Autodesk Fusion 360 part; units mm, degrees
note: some values were not read from the file. Set by a fixed rule: which sketch regions a step uses.
(part 7 of 7)
  spline S19 degree 5 poles (3.4043, 3.4422) (3.4043, 3.4423) (3.4044, 3.4423) (3.4045, 3.4425) (3.4047, 3.4427) (3.405, 3.443) (3.4054, 3.4433) (3.4058, 3.4437) (3.4063, 3.4441) (3.4068, 3.4446) (3.4073, 3.4451) (3.4079, 3.4457) (3.4085, 3.4462) (3.4092, 3.4469) (3.41, 3.4475) (3.4107, 3.4482) (3.4116, 3.449) (3.4124, 3.4497) (3.4134, 3.4505) (3.4143, 3.4514) (3.4153, 3.4523) (3.4164, 3.4532) (3.4175, 3.4541) (3.4187, 3.4551) (3.4199, 3.4561) (3.4211, 3.4571) (3.4224, 3.4582) (3.4237, 3.4593) (3.4251, 3.4604) (3.4265, 3.4616) (3.428, 3.4628) (3.4295, 3.464) (3.4311, 3.4652) (3.4327, 3.4665) (3.4344, 3.4678) (3.4361, 3.4691) (3.4378, 3.4705) (3.4396, 3.4718) (3.4414, 3.4732) (3.4433, 3.4747) (3.4453, 3.4761) (3.4472, 3.4776) (3.4492, 3.4791) (3.4513, 3.4806) (3.4534, 3.4821) (3.4556, 3.4837) (3.4577, 3.4852) (3.46, 3.4868) (3.4623, 3.4885) (3.4646, 3.4901) (3.467, 3.4918) (3.4694, 3.4934) (3.4718, 3.4951) (3.4743, 3.4968) (3.4769, 3.4986) (3.4795, 3.5003) (3.4821, 3.5021) (3.4848, 3.5039) (3.4875, 3.5057) (3.4903, 3.5075) (3.4931, 3.5093) (3.4959, 3.5112) (3.4988, 3.513) (3.5018, 3.5149) (3.5047, 3.5168) (3.5078, 3.5187) (3.5108, 3.5206) (3.5139, 3.5225) (3.5171, 3.5244) (3.5203, 3.5264) (3.5235, 3.5284) (3.5268, 3.5303) (3.5301, 3.5323) (3.5335, 3.5343) (3.5369, 3.5363) (3.5403, 3.5383) (3.5438, 3.5404) (3.5473, 3.5424) (3.5509, 3.5444) (3.5545, 3.5465) (3.5582, 3.5486) (3.5619, 3.5506) (3.5656, 3.5527) (3.5694, 3.5548) (3.5732, 3.5569) (3.577, 3.559) (3.5809, 3.5611) (3.5849, 3.5632) (3.5889, 3.5653) (3.5929, 3.5674) (3.5969, 3.5696) (3.6011, 3.5717) (3.6052, 3.5738) (3.6094, 3.576) (3.6136, 3.5781) (3.6179, 3.5803) (3.6222, 3.5824) (3.6265, 3.5846) (3.6309, 3.5868) (3.6353, 3.5889) (3.6398, 3.5911) (3.6443, 3.5933) (3.6488, 3.5954) (3.6534, 3.5976) (3.658, 3.5998) (3.6627, 3.602) (3.6674, 3.6041) (3.6721, 3.6063) (3.6769, 3.6085) (3.6817, 3.6107) (3.6865, 3.6129) (3.6914, 3.615) (3.6964, 3.6172) (3.7013, 3.6194) (3.7063, 3.6216) (3.7114, 3.6238) (3.7165, 3.6259) (3.7216, 3.6281) (3.7267, 3.6303) (3.7319, 3.6324) (3.7372, 3.6346) (3.7424, 3.6368) (3.7477, 3.6389) (3.7531, 3.6411) (3.7585, 3.6433) (3.7639, 3.6454) (3.7693, 3.6476) (3.7748, 3.6497) (3.7803, 3.6518) (3.7859, 3.654) (3.7915, 3.6561) (3.7972, 3.6582) (3.8028, 3.6604) (3.8085, 3.6625) (3.8143, 3.6646) (3.8201, 3.6667) (3.8259, 3.6688) (3.8317, 3.6709) (3.8376, 3.673) (3.8436, 3.675) (3.8495, 3.6771) (3.8555, 3.6792) (3.8615, 3.6812) (3.8676, 3.6833) (3.8737, 3.6853) (3.8799, 3.6874) (3.886, 3.6894) (3.8922, 3.6914) (3.8985, 3.6934) (3.9048, 3.6954) (3.9111, 3.6974) (3.9174, 3.6994) (3.9238, 3.7014) (3.9302, 3.7034) (3.9366, 3.7053) (3.9431, 3.7073) (3.9496, 3.7092) (3.9562, 3.7112) (3.9628, 3.7131) (3.9694, 3.715) (3.976, 3.7169) (3.9827, 3.7188) (3.9894, 3.7207) (3.9962, 3.7225) (4.003, 3.7244) (4.0098, 3.7262) (4.0166, 3.7281) (4.0235, 3.7299) (4.0304, 3.7317) (4.0374, 3.7335) (4.0444, 3.7353) (4.0514, 3.7371) (4.0584, 3.7388) (4.0655, 3.7406) (4.0726, 3.7423) (4.0797, 3.744) (4.0869, 3.7457) (4.0941, 3.7474) (4.1013, 3.7491) (4.1086, 3.7508) (4.1159, 3.7524) (4.1232, 3.7541) (4.1306, 3.7557) (4.138, 3.7573) (4.1454, 3.7589) (4.1528, 3.7605) (4.1603, 3.7621) (4.1678, 3.7636) (4.1754, 3.7652) (4.1829, 3.7667) (4.1905, 3.7682) (4.1982, 3.7697) (4.2058, 3.7712) (4.2135, 3.7727) (4.2212, 3.7741) (4.229, 3.7755) (4.2368, 3.7769) (4.2446, 3.7783) (4.2524, 3.7797) (4.2603, 3.7811) (4.2682, 3.7825) (4.2761, 3.7838) (4.2841, 3.7851) (4.2921, 3.7864) (4.3001, 3.7877) (4.3081, 3.789) (4.3162, 3.7902) (4.3243, 3.7914) (4.3324, 3.7926) (4.3406, 3.7938) (4.3488, 3.795) (4.357, 3.7962) (4.3652, 3.7973) (4.3735, 3.7984) (4.3818, 3.7995) (4.3901, 3.8006) (4.3984, 3.8017) (4.4068, 3.8027) (4.4152, 3.8038) (4.4236, 3.8048) (4.4321, 3.8058) (4.4406, 3.8067) (4.4491, 3.8077) (4.4576, 3.8086) (4.4662, 3.8095) (4.4748, 3.8104) (4.4834, 3.8113) (4.4921, 3.8122) (4.5007, 3.813) (4.5094, 3.8138) (4.5181, 3.8146) (4.5269, 3.8154) (4.5357, 3.8161) (4.5445, 3.8169) (4.5533, 3.8176) (4.5621, 3.8183) (4.571, 3.8189) (4.5799, 3.8196) (4.5888, 3.8202) (4.5978, 3.8208) (4.6067, 3.8214) (4.6139, 3.8218) (4.6194, 3.8222) (4.623, 3.8224) (4.6248, 3.8225) knots 0 0 0 0 0 0 0.00416667 0.00833333 0.0125 0.01666667 0.02083333 0.025 0.02916667 0.03333333 0.0375 0.04166667 0.04583333 0.05 0.05416667 0.05833333 0.0625 0.06666667 0.07083333 0.075 0.07916667 0.08333333 0.0875 0.09166667 0.09583333 0.1 0.10416667 0.10833333 0.1125 0.11666667 0.12083333 0.125 0.12916667 0.13333333 0.1375 0.14166667 0.14583333 0.15 0.15416667 0.15833333 0.1625 0.16666667 0.17083333 0.175 0.17916667 0.18333333 0.1875 0.19166667 0.19583333 0.2 0.20416667 0.20833333 0.2125 0.21666667 0.22083333 0.225 0.22916667 0.23333333 0.2375 0.24166667 0.24583333 0.25 0.25416667 0.25833333 0.2625 0.26666667 0.27083333 0.275 0.27916667 0.28333333 0.2875 0.29166667 0.29583333 0.3 0.30416667 0.30833333 0.3125 0.31666667 0.32083333 0.325 0.32916667 0.33333333 0.3375 0.34166667 0.34583333 0.35 0.35416667 0.35833333 0.3625 0.36666667 0.37083333 0.375 0.37916667 0.38333333 0.3875 0.39166667 0.39583333 0.4 0.40416667 0.40833333 0.4125 0.41666667 0.42083333 0.425 0.42916667 0.43333333 0.4375 0.44166667 0.44583333 0.45 0.45416667 0.45833333 0.4625 0.46666667 0.47083333 0.475 0.47916667 0.48333333 0.4875 0.49166667 0.49583333 0.5 0.50416667 0.50833333 0.5125 0.51666667 0.52083333 0.525 0.52916667 0.53333333 0.5375 0.54166667 0.54583333 0.55 0.55416667 0.55833333 0.5625 0.56666667 0.57083333 0.575 0.57916667 0.58333333 0.5875 0.59166667 0.59583333 0.6 0.60416667 0.60833333 0.6125 0.61666667 0.62083333 0.625 0.62916667 0.63333333 0.6375 0.64166667 0.64583333 0.65 0.65416667 0.65833333 0.6625 0.66666667 0.67083333 0.675 0.67916667 0.68333333 0.6875 0.69166667 0.69583333 0.7 0.70416667 0.70833333 0.7125 0.71666667 0.72083333 0.725 0.72916667 0.73333333 0.7375 0.74166667 0.74583333 0.75 0.75416667 0.75833333 0.7625 0.76666667 0.77083333 0.775 0.77916667 0.78333333 0.7875 0.79166667 0.79583333 0.8 0.80416667 0.80833333 0.8125 0.81666667 0.82083333 0.825 0.82916667 0.83333333 0.8375 0.84166667 0.84583333 0.85 0.85416667 0.85833333 0.8625 0.86666667 0.87083333 0.875 0.87916667 0.88333333 0.8875 0.89166667 0.89583333 0.9 0.90416667 0.90833333 0.9125 0.91666667 0.92083333 0.925 0.92916667 0.93333333 0.9375 0.94166667 0.94583333 0.95 0.95416667 0.95833333 0.9625 0.96666667 0.97083333 0.975 0.97916667 0.98333333 0.9875 0.99166667 0.99583333 1 1 1 1 1 1
  line L38 (3.4039, 3.4418) -> (3.4043, 3.4422)
  line L39 (3.4039, 3.4418) -> (2.6369, 2.6663)
  circle A20 centre (0, 0) radius 4.8
  dimension "d12" = 9.6
  constraint concentric A0 A20
  measures "d12" diameter of A20
extrude "돌출4" add sketch "스케치2 (2)" along normal blind 10 contours A0 L0 L3 A2 L4 L7 A4 L8 L11 A6 L12 L15 A8 L16 L19 A10 L20 L23 A12 L24 L27 A14 L28 L31 A16 L32 L35 A18 L36 L39 A20 | A0 L0 L39 A20 | L35 A18 L36 A20 | L3 A2 L4 A20 | L7 A4 L8 A20 | L31 A16 L32 A20 | L11 A6 L12 A20 | L27 A14 L28 A20 | L15 A8 L16 A20 | L23 A12 L24 A20 | L19 A10 L20 A20 bodies 1 in component "Component"
component "Component" placed x (1, 0, 0) y (0, 1, 0) z (0, 0, 1) at (0, 0, 0)
